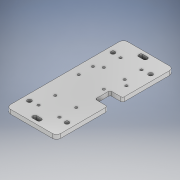
# Autodesk Inventor part: Y-Axis_front_plate_bottom
Saved by Autodesk Inventor 2021.3 (Build 253353000, 353)
## iProperties
Created: 2021-04-15
Part Number: Y-Axis_front_plate_bottom
Material: Generic
Document SubType Name: Modeling
Designer: Fabijan_Sven
Density: 1 g/cm^3
Appearance: Aluminum - Polished
Author: Fabijan_Sven
Autodesk Inventor part; units mm, degrees
ref_plane "YZ Plane" through (0, 0, 0) normal (1, 0, 0) x (0, 1, 0)
ref_plane "XZ Plane" through (0, 0, 0) normal (0, 1, 0) x (-1, 0, 0)
ref_plane "XY Plane" through (0, 0, 0) normal (0, 0, 1) x (1, 0, 0)
sketch "Sketch1" plane through (0, 0, 0) normal (0, 1, 0) x (-1, 0, 0)
  line L0 (0, 0) -> (60, 0)
  line L1 (60, 0) -> (60, -140)
  line L2 (60, -140) -> (0, -140)
  line L3 (0, -140) -> (0, 0)
  line L4 (30, -20.8594) -> (30, -183.1932) construction
  line L5 (42.5, -21.7206) -> (42.5, -191.0157) construction
  line L6 (17.5, -21.7206) -> (17.5, -184.1979) construction
  circle A0 centre (42.5, -21) radius 1.5
  circle A1 centre (42.5, -41) radius 1.5
  circle A2 centre (42.5, -99) radius 1.5
  circle A3 centre (42.5, -119) radius 1.5
  circle A4 centre (17.5, -99) radius 1.5
  circle A5 centre (17.5, -119) radius 1.5
  circle A6 centre (17.5, -41) radius 1.5
  circle A7 centre (17.5, -21) radius 1.5
  dimension "d0" = 140
  dimension "d1" = 60
  dimension "d2" = 30
  dimension "d3" = 12.5
  dimension "d4" = 12.5
  dimension "d5" = 3
  dimension "d6" = 3
  dimension "d7" = 3
  dimension "d8" = 3
  dimension "d9" = 3
  dimension "d10" = 3
  dimension "d11" = 3
  dimension "d12" = 3
  dimension "d13" = 20
  dimension "d14" = 20
  dimension "d15" = 20
  dimension "d16" = 20
  dimension "d17" = 21
  dimension "d18" = 21
  dimension "d19" = 21
  dimension "d20" = 21
  constraints: 14 end point, 8 centre point, 8 point on line, 3 vertical, 2 parallel, 1 horizontal, 1 perpendicular
  measures "d0" distance of L0.end L1.end
  measures "d1" distance of L1.end L2.end
  measures "d2" distance between parallel lines of L4 L1
  measures "d3" distance between parallel lines of L5 L4
  measures "d4" distance between parallel lines of L6 L4
  measures "d5" diameter of A0
  measures "d6" diameter of A1
  measures "d7" diameter of A2
  measures "d8" diameter of A3
  measures "d9" diameter of A4
  measures "d10" diameter of A5
  measures "d11" diameter of A6
  measures "d12" diameter of A7
  measures "d13" distance of A1.centre A0.centre
  measures "d14" distance of A6.centre A7.centre
  measures "d15" distance of A3.centre A2.centre
  measures "d16" distance of A5.centre A4.centre
  measures "d17" distance from line of L0 A0.centre
  measures "d18" distance from line of L0 A7.centre
  measures "d19" distance from line of L2 A3.centre
  measures "d20" distance from line of A5.centre L2
extrude "Extrusion1" add sketch "Sketch1" along normal blind 5
sketch "Sketch2" plane through (0, 0, 0) normal (0, -1, 0) x (1, 0, 0)
  circle A0 centre (-7.5, -20) radius 2.5
  circle A1 centre (-7.5, -120) radius 2.5
  circle A2 centre (-52.5, -20) radius 2.5
  circle A3 centre (-52.5, -120) radius 2.5
  line L0 (-60, 0) -> (0, 0) projected
  line L1 (0, 0) -> (0, -140) projected
  line L2 (-60, -140) -> (-60, 0) projected
  line L3 (0, -140) -> (-60, -140) projected
  dimension "d23" = 5
  dimension "d24" = 5
  dimension "d25" = 5
  dimension "d26" = 5
  dimension "d27" = 20
  dimension "d28" = 7.5
  dimension "d29" = 20
  dimension "d30" = 7.5
  dimension "d31" = 20
  dimension "d32" = 7.5
  dimension "d33" = 20
  dimension "d34" = 7.5
  constraints: 4 centre point
  measures "d23" diameter of A0
  measures "d24" diameter of A1
  measures "d25" diameter of A2
  measures "d26" diameter of A3
  measures "d27" distance from line of L0 A0.centre
  measures "d28" distance from line of A0.centre L1
  measures "d29" distance from line of L0 A2.centre
  measures "d30" distance from line of L2 A2.centre
  measures "d31" distance from line of L3 A1.centre
  measures "d32" distance from line of L1 A1.centre
  measures "d33" distance from line of A3.centre L3
  measures "d34" distance from line of L2 A3.centre
extrude "Extrusion2" cut sketch "Sketch2" against normal blind 10 contours A0 | A1 | A2 | A3
sketch "Sketch3" plane through (0, 0, 0) normal (0, -1, 0) x (1, 0, 0)
  line L0 (-25, -4) -> (-35, -4)
  line L1 (-35, -4) -> (-35, -9)
  line L2 (-35, -9) -> (-25, -9)
  line L3 (-25, -9) -> (-25, -4)
  line L4 (9.3646, -70) -> (-76.8402, -70) construction
  line L5 (-60, 0) -> (0, 0) projected
  line L6 (0, 0) -> (0, -140) projected
  line L7 (-25, -136) -> (-35, -136)
  line L8 (-35, -136) -> (-35, -131)
  line L9 (-35, -131) -> (-25, -131)
  line L10 (-25, -131) -> (-25, -136)
  dimension "d40" = 70
  dimension "d41" = 10
  dimension "d42" = 4
  dimension "d43" = 5
  dimension "d44" = 25
  constraints: 18 end point, 4 symmetric about line, 2 horizontal, 2 parallel, 1 perpendicular
  measures "d40" distance between parallel lines of L5 L4
  measures "d41" distance of L0.start L0.end
  measures "d42" distance between parallel lines of L5 L0
  measures "d43" distance of L2.end L0.start
  measures "d44" distance between parallel lines of L3 L6
extrude "Extrusion3" cut sketch "Sketch3" against normal blind 10
fillet "Fillet2" radius 5 4 edges at (-60, 2.5, 0) (-60, 2.5, -140) (0, 2.5, -140) (0, 2.5, 0)
sketch "Sketch4" plane through (0, 5, 0) normal (0, 1, 0) x (1, 0, 0)
  circle A0 centre (-50, 76.5) radius 1.5
  circle A1 centre (-50, 93.5) radius 1.5
  circle A2 centre (-20, 76.5) radius 1.5
  circle A3 centre (-10, 93.5) radius 1.5
  line L0 (-5, 140) -> (-55, 140) projected
  line L1 (-60, 135) -> (-60, 5) projected
  line L2 (0, 5) -> (0, 135) projected
  point P0 (0, 0)
  dimension "d49" = 3
  dimension "d50" = 3
  dimension "d51" = 3
  dimension "d52" = 3
  dimension "d53" = 46.5
  dimension "d54" = 46.5
  dimension "d55" = 63.5
  dimension "d56" = 63.5
  dimension "d57" = 10
  dimension "d59" = 10
  dimension "d71" = 10
  dimension "d72" = 20
  constraints: 4 centre point
  measures "d49" diameter of A0
  measures "d50" diameter of A2
  measures "d51" diameter of A1
  measures "d52" diameter of A3
  measures "d53" distance from line of A1.centre L0
  measures "d54" distance from line of L0 A3.centre
  measures "d55" distance from line of A0.centre L0
  measures "d56" distance from line of A2.centre L0
  measures "d57" distance from line of L1 A0.centre
  measures "d59" distance from line of L1 A1.centre
  measures "d71" distance from line of L2 A3.centre
  measures "d72" distance from line of L2 A2.centre
extrude "Extrusion4" cut sketch "Sketch4" against normal blind 10
sketch "Sketch5" plane through (0, 0, 0) normal (0, -1, 0) x (1, 0, 0)
  line L0 (59.7124, -61) -> (87.7124, -61) projected
  line L1 (87.7124, -79) -> (59.7124, -79) projected
  line L2 (5, -61) -> (-15, -61)
  line L3 (-15, -61) -> (-15, -79)
  line L4 (-15, -79) -> (5, -79)
  line L5 (5, -79) -> (5, -61)
  line L6 (0, -5) -> (0, -135) projected
  point P0 (0, 0)
  dimension "d66" = 15
  dimension "d67" = 5
  constraints: 8 end point, 2 collinear, 2 parallel, 1 horizontal, 1 perpendicular
  measures "d66" distance between parallel lines of L3 L6
  measures "d67" distance between parallel lines of L6 L5
extrude "Extrusion5" cut sketch "Sketch5" against normal blind 10
fillet "Fillet3" radius 2 4 edges at (0, 2.5, -79) (0, 2.5, -61) (-15, 2.5, -79) (-15, 2.5, -61)
fillet "Fillet4" radius 2 8 edges at (-25, 2.5, -9) (-25, 2.5, -4) (-35, 2.5, -4) (-35, 2.5, -9) (-35, 2.5, -136) (-35, 2.5, -131) (-25, 2.5, -131) (-25, 2.5, -136)
equation "\"d2\" = 0.5 * d1"
equation "\"d4\" = d3"
equation "\"d6\" = d5"
equation "\"d7\" = d5"
equation "\"d8\" = d5"
equation "\"d9\" = d5"
equation "\"d10\" = d5"
equation "\"d11\" = d5"
equation "\"d12\" = d5"
equation "\"d14\" = d13"
equation "\"d15\" = d13"
equation "\"d16\" = d13"
equation "\"d18\" = d17"
equation "\"d19\" = d17"
equation "\"d20\" = d17"
equation "\"d29\" = d27"
equation "\"d30\" = d28"
equation "\"d31\" = d27"
equation "\"d32\" = d28"
equation "\"d33\" = d27"
equation "\"d34\" = d28"
equation "\"d50\" = d49"
equation "\"d51\" = d49"
equation "\"d52\" = d49"
body "Solid1"
